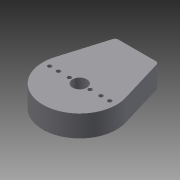
# Autodesk Inventor part: encoder
Saved by Autodesk Inventor 2015 (Build 190159000, 159)
## iProperties
Created: 2015-12-08
Part Number: encoder
Material: Generic
Document SubType Name: Modeling
Designer: boztalay
Density: 1 g/cm^3
Appearance: Default
Author: boztalay
Autodesk Inventor part; units mm, degrees
ref_plane "YZ Plane" through (0, 0, 0) normal (1, 0, 0) x (0, 1, 0)
ref_plane "XZ Plane" through (0, 0, 0) normal (0, 1, 0) x (-1, 0, 0)
ref_plane "XY Plane" through (0, 0, 0) normal (0, 0, 1) x (1, 0, 0)
sketch "Sketch1" plane through (0, 0, 0) normal (0, 1, 0) x (-1, 0, 0)
  arc A0 (27.0056, -8.0993) -> (-27.0056, -8.0993) centre (0, 0) ccw
  line L0 (0, -43.942) -> (14.366, -43.942)
  line L1 (-14.366, -43.942) -> (0, -43.942)
  line L2 (0, 15.1299) -> (0, -95.843) construction
  line L3 (33.8234, 0) -> (-34.0336, 0) construction
  line L4 (16.256, 0) -> (16.256, -43.942) construction
  line L5 (16.7989, -42.1317) -> (27.0056, -8.0993)
  line L6 (-16.7989, -42.1317) -> (-27.0056, -8.0993)
  circle A1 centre (0, 0) radius 5.5372
  arc A2 (14.366, -43.942) -> (16.7989, -42.1317) centre (14.366, -41.402) ccw
  arc A3 (-16.7989, -42.1317) -> (-14.366, -43.942) centre (-14.366, -41.402) ccw
  circle A4 centre (7.9375, 0) radius 1.524
  line L7 (0, 0) -> (7.9375, 0) construction
  circle A5 centre (-7.9375, 0) radius 1.524
  line L8 (0, 0) -> (-7.9375, 0) construction
  circle A6 centre (16.256, 0) radius 1.524
  line L9 (0, 0) -> (16.256, 0) construction
  circle A7 centre (-16.256, 0) radius 1.524
  line L10 (0, 0) -> (-16.256, 0) construction
  circle A8 centre (23.0124, 0) radius 1.524
  line L11 (0, 0) -> (23.0124, 0) construction
  circle A9 centre (-23.0124, 0) radius 1.524
  line L12 (0, 0) -> (-23.0124, 0) construction
  point P0 (-16.256, -43.942)
  dimension "d0" = 56.388
  dimension "d4" = 16.256
  dimension "d5" = 16.256
  dimension "d6" = 43.942
  dimension "d7" = 11.0744
  dimension "d8" = 2.54
  dimension "d9" = 3.048
  dimension "d10" = 7.9375
  dimension "d12" = 3.048
  dimension "d13" = 16.256
  dimension "d15" = 3.048
  dimension "d16" = 23.0124
  constraints: 26 end point, 10 centre point, 9 point on line, 6 horizontal, 6 point on circle, 6 tangent, 3 symmetric about line, 3 vertical, 2 coincident, 2 collinear, 1 equal radius, 3 other
  measures "d0" diameter of A0
  measures "d4" distance of L0.start L4.end
  measures "d5" distance of L0.start point (-16.256, -43.942)
  measures "d6" distance of L4.end L4.start
  measures "d7" diameter of A1
  measures "d8" radius of A2
  measures "d9" diameter of A4
  measures "d10" distance of L7.start L7.end
  measures "d12" diameter of A6
  measures "d13" distance of L7.start L9.end
  measures "d15" diameter of A8
  measures "d16" distance of L7.start L11.end
extrude "Extrusion1" add sketch "Sketch1" along normal blind 16.51
body "Solid1"
